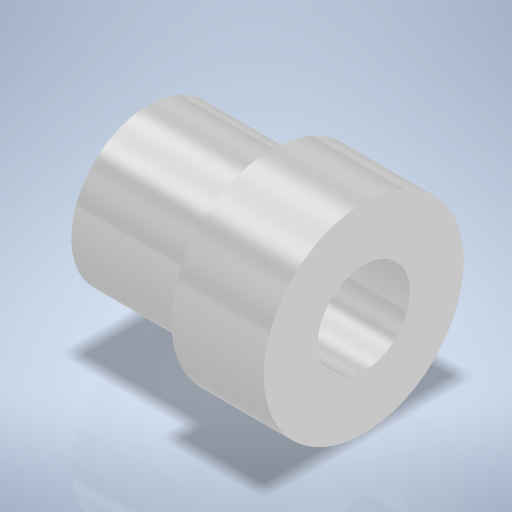
# Autodesk Inventor part: 10167ipt
Saved by Autodesk Inventor 2024 (Build 280153000, 153)
## iProperties
Created: 2024-07-12
Part Number: 10167ipt
Material: Aluminum 6061-AHC
Document SubType Name: Modeling
Designer: ffogue
Density: 2.7 g/cm^3
Appearance: Aluminium - dunkel
Author: ffogue
Autodesk Inventor part; units mm, degrees
ref_plane "YZ Plane" through (0, 0, 0) normal (1, 0, 0) x (0, 1, 0)
ref_plane "XZ Plane" through (0, 0, 0) normal (0, 1, 0) x (-1, 0, 0)
ref_plane "XY Plane" through (0, 0, 0) normal (0, 0, 1) x (1, 0, 0)
sketch "Skizze1" plane through (0, 0, 0) normal (0, 1, 0) x (-1, 0, 0)
  line L0 (0, 0) -> (0, 5)
  line L1 (0, 5) -> (-8, 5)
  line L2 (-8, 5) -> (-8, 6.5)
  line L3 (-8, 6.5) -> (-14, 6.5)
  line L4 (-14, 6.5) -> (-14, 0)
  line L5 (-14, 0) -> (0, 0)
  dimension "d0" = 6
  dimension "d1" = 8
  dimension "d2" = 10
  dimension "d3" = 13
  constraints: 12 end point, 5 perpendicular, 1 vertical
  measures "d0" distance between parallel lines of L4 L2
  measures "d1" distance between parallel lines of L2 L0
  measures "d2" diameter of L1 L5
  measures "d3" diameter of L3 L5
revolve "Umdrehung1" add sketch "Skizze1" angle 360 about axis through (14, 0, 0) along (-1, 0, 0)
sketch "Skizze2" plane through (0, 0, 0) normal (-1, 0, 0) x (0, 0, 1)
  circle A0 centre (0, 0) radius 5 projected
  point P0 (0, 0)
  constraints: 1 coincident
hole "Bohrung1" at (0, 0, 0) direction (1, 0, 0) diameter 6 depth 14
